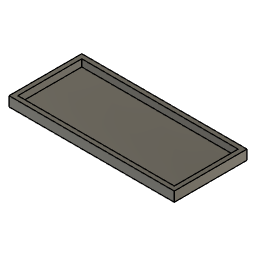
Frame_bottom (Autodesk Fusion 360 design; units mm, degrees)
Autodesk Fusion 360 part; units mm, degrees
sketch "Sketch1" plane through (0, 0, 0) normal (0, 0, 1) x (1, 0, 0)
  line L0 (0, 0) -> (187.5, 0)
  line L1 (187.5, 0) -> (187.5, 82.5)
  line L2 (187.5, 82.5) -> (0, 82.5)
  line L3 (0, 82.5) -> (0, 0)
  dimension "d1" = 187.5
  dimension "d2" = 82.5
  constraint horizontal L0
  constraint vertical L1
  constraint horizontal L2
  constraint vertical L3
  constraint coincident L0.start L3.end
  measures "d1" distance of L0.start L0.end
  measures "d2" distance of L0.start L2.end
extrude "Extrude1" add sketch "Sketch1" along normal blind 3
sketch "Sketch2" plane through (0, 0, 3) normal (0, 0, 1) x (-1, 0, 0)
  line L0 (0, -82.5) -> (0, 0)
  line L1 (0, 0) -> (-187.5, 0)
  line L2 (-187.5, 0) -> (-187.5, -82.5)
  line L3 (-187.5, -82.5) -> (0, -82.5)
  line L4 (-5, -5) -> (-182.5, -5)
  line L5 (-182.5, -5) -> (-182.5, -77.5)
  line L6 (-182.5, -77.5) -> (-5, -77.5)
  line L7 (-5, -77.5) -> (-5, -5)
  dimension "d5" = -5
extrude "Extrude2" add sketch "Sketch2" along normal blind 8
